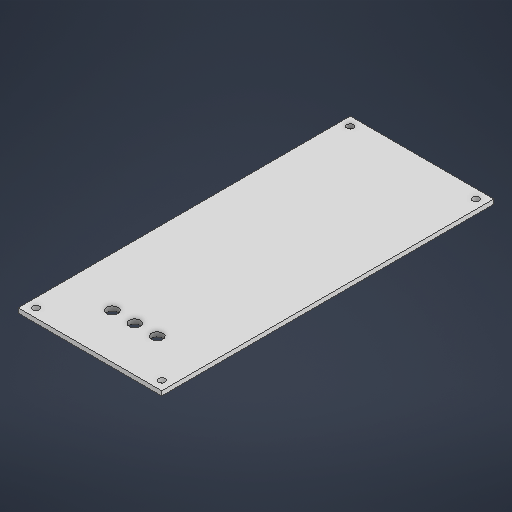
# Autodesk Inventor part: kotelo_kansi
Saved by Autodesk Inventor 2026 (Build 300175000, 175)
## iProperties
Created: 2026-01-15
Part Number: kotelo_kansi
Material: Generic
Document SubType Name: Modeling
Designer: toni.hatala
Density: 1 g/cm^3
Appearance: Default
Author: toni.hatala
Autodesk Inventor part; units mm, degrees
ref_plane "YZ Plane" through (0, 0, 0) normal (1, 0, 0) x (0, 1, 0)
ref_plane "XZ Plane" through (0, 0, 0) normal (0, 1, 0) x (-1, 0, 0)
ref_plane "XY Plane" through (0, 0, 0) normal (0, 0, 1) x (1, 0, 0)
sketch "Sketch2" plane through (0, 0, 0) normal (0, 1, 0) x (-1, 0, 0)
  line L0 (0, 0) -> (64, 0)
  line L1 (64, 0) -> (64, -148)
  line L2 (64, -148) -> (0, -148)
  line L3 (0, -148) -> (0, 0)
  dimension "d0" = 64
  dimension "d1" = 148
  constraints: 8 end point, 2 parallel, 1 horizontal, 1 perpendicular
  measures "d0" distance of L1.end L2.end
  measures "d1" distance of L0.end L1.end
extrude "Extrusion1" add sketch "Sketch2" along normal blind 2
sketch "Sketch3" plane through (0, 2, 0) normal (0, 1, 0) x (1, 0, 0)
  circle A0 centre (-4, 4) radius 1.5
  circle A1 centre (-60, 4) radius 1.5
  circle A2 centre (-60, 144) radius 1.5
  circle A3 centre (-4, 144) radius 1.5
  line L0 (0, 0) -> (0, 148) projected
  line L1 (-64, 0) -> (0, 0) projected
  line L2 (-64, 148) -> (-64, 0) projected
  line L3 (0, 148) -> (-64, 148) projected
  point P0 (0, 0.5)
  point P1 (0, 147.5)
  point P2 (-63.5, 0)
  point P3 (-0.5, 0)
  point P4 (-64, 147.5)
  point P5 (-64, 0.5)
  point P6 (-0.5, 148)
  point P7 (-63.5, 148)
  dimension "d10" = 3
  dimension "d11" = 3
  dimension "d12" = 3
  dimension "d13" = 3
  dimension "d14" = 4
  dimension "d15" = 4
  dimension "d16" = 4
  dimension "d17" = 4
  dimension "d18" = 4
  dimension "d19" = 4
  dimension "d20" = 4
  dimension "d21" = 4
  constraints: 4 centre point
  measures "d10" diameter of A0
  measures "d11" diameter of A1
  measures "d12" diameter of A2
  measures "d13" diameter of A3
  measures "d14" distance from line of L0 A0.centre
  measures "d15" distance from line of L1 A0.centre
  measures "d16" distance from line of L2 A1.centre
  measures "d17" distance from line of L1 A1.centre
  measures "d18" distance from line of L2 A2.centre
  measures "d19" distance from line of L3 A2.centre
  measures "d20" distance from line of L3 A3.centre
  measures "d21" distance from line of L0 A3.centre
extrude "Extrusion2" cut sketch "Sketch3" against normal blind 2 contours A0 | A1 | A2 | A3
sketch "Sketch4" plane through (0, 2, 0) normal (0, 1, 0) x (1, 0, 0)
  circle A0 centre (-22, 20) radius 2.5
  circle A1 centre (-32, 20) radius 2.5
  circle A2 centre (-42, 20) radius 2.5
  line L0 (0, 0) -> (0, 148) projected
  line L1 (-64, 0) -> (0, 0) projected
  point P0 (0, 0.5)
  point P1 (0, 147.5)
  point P2 (-63.5, 0)
  point P3 (-0.5, 0)
  point P4 (-32, 0)
  dimension "d24" = 5
  dimension "d25" = 5
  dimension "d26" = 5
  dimension "d28" = 32
  dimension "d29" = 10
  dimension "d30" = 10
  dimension "d31" = 20
  constraints: 3 centre point, 1 midpoint
  measures "d24" diameter of A0
  measures "d25" diameter of A1
  measures "d26" diameter of A2
  measures "d28" distance from line of L0 A1.centre
  measures "d29" distance of A1.centre A2.centre
  measures "d30" distance of A0.centre A1.centre
  measures "d31" distance of point (-32, 0) A1.centre
extrude "Extrusion3" cut sketch "Sketch4" against normal blind 2
body "Solid1"
